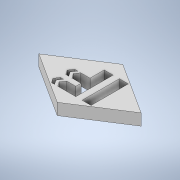
# Autodesk Inventor part: TeamIF
Saved by Autodesk Inventor 2020 (Build 240168000, 168)
## iProperties
Created: 2020-07-04
Part Number: TeamIF
Material: Generic
Document SubType Name: Modeling
Designer: maple
Density: 1 g/cm^3
Appearance: Default
Author: maple
Autodesk Inventor part; units mm, degrees
ref_plane "YZ Plane" through (0, 0, 0) normal (1, 0, 0) x (0, 1, 0)
ref_plane "XZ Plane" through (0, 0, 0) normal (0, 1, 0) x (-1, 0, 0)
ref_plane "XY Plane" through (0, 0, 0) normal (0, 0, 1) x (1, 0, 0)
sketch "Sketch1" plane through (0, 0, 0) normal (0, 1, 0) x (-1, 0, 0)
  line L0 (0, 0) -> (361.1993, 0) construction
  line L1 (361.1993, 0) -> (361.1993, -361.1993) construction
  line L2 (361.1993, -361.1993) -> (0, -361.1993) construction
  line L3 (0, -361.1993) -> (0, 0) construction
  constraints: 2 other
sketch "Sketch2" plane through (0, 0, 0) normal (0, 1, 0) x (-1, 0, 0)
  line L0 (0, -180.5996) -> (11.43, -180.5996)
  line L1 (11.43, -180.5996) -> (180.5997, -72.009)
  line L2 (180.5997, -289.1903) -> (11.43, -180.5996)
  line L3 (361.1993, -180.5996) -> (349.7693, -180.5996)
  line L4 (349.7693, -180.5996) -> (180.5997, -72.009)
  line L5 (180.5997, -289.1903) -> (349.7693, -180.5996)
  line L6 (115.508, -119.0216) -> (145.1807, -119.0216)
  line L7 (145.1807, -119.0216) -> (145.1807, -242.5337)
  line L8 (145.1807, -242.5337) -> (115.508, -242.5337)
  line L9 (115.508, -242.5337) -> (115.508, -119.0216)
  line L10 (165.8332, -118.9647) -> (165.8332, -242.4769)
  line L11 (165.8332, -242.4769) -> (195.5355, -242.4769)
  line L12 (195.5355, -242.4769) -> (195.5355, -195.5556)
  line L13 (195.5355, -195.5556) -> (225.8549, -195.5556)
  line L14 (225.8549, -195.5556) -> (236.0754, -180.9592)
  line L15 (236.0754, -180.9592) -> (225.5562, -165.8753)
  line L16 (225.5562, -165.8753) -> (195.5355, -165.8753)
  line L17 (195.5355, -165.8753) -> (195.5355, -148.6741)
  line L18 (195.5355, -148.6741) -> (225.5562, -148.6741)
  line L19 (225.5562, -148.6741) -> (235.7293, -133.6668)
  line L20 (235.7293, -133.6668) -> (225.8549, -118.9647)
  line L21 (225.8549, -118.9647) -> (165.8332, -118.9647)
  line L22 (236.3576, -118.9647) -> (246.1353, -118.9647)
  line L23 (246.1353, -118.9647) -> (256.2661, -133.6668)
  line L24 (236.0628, -148.731) -> (246.0969, -148.731)
  line L25 (246.0969, -148.731) -> (256.2661, -133.6668)
  line L26 (236.3576, -118.9647) -> (246.2319, -133.6668)
  line L27 (236.0628, -148.731) -> (246.2319, -133.6668)
  line L28 (236.3576, -165.8976) -> (246.1353, -165.8976)
  line L29 (246.1353, -165.8976) -> (256.2661, -180.5996)
  line L30 (236.0628, -195.6639) -> (246.0969, -195.6639)
  line L31 (246.0969, -195.6639) -> (256.2661, -180.5996)
  line L32 (236.3576, -165.8976) -> (246.2319, -180.5996)
  line L33 (236.0628, -195.6639) -> (246.2319, -180.5996)
  point P0 (0, 0)
  dimension "d1" = 11.43
  dimension "d3" = 11.43
  dimension "d4" = 125
  dimension "d5" = 90
  constraints: 68 end point, 7 parallel, 6 horizontal, 4 perpendicular
  measures "d1" distance of L0.start L0.end
  measures "d3" distance of L3.start L3.end
  measures "d4" angle of L14 L13
  measures "d5" angle of L17 L18
extrude "Extrusion1" add sketch "Sketch2" along normal blind 38.1
body "Solid1"
